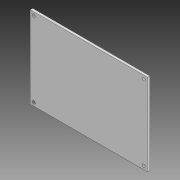
# Autodesk Inventor part: Motherboard
Saved by Autodesk Inventor 2020 (Build 240168000, 168)
## iProperties
Created: 2021-06-02
Part Number: Motherboard
Material: Generic
Document SubType Name: Modeling
Designer: DDeGo
Density: 1 g/cm^3
Appearance: Default
Author: DDeGo
Autodesk Inventor part; units mm, degrees
ref_plane "YZ Plane" through (0, 0, 0) normal (1, 0, 0) x (0, 1, 0)
ref_plane "XZ Plane" through (0, 0, 0) normal (0, 1, 0) x (-1, 0, 0)
ref_plane "XY Plane" through (0, 0, 0) normal (0, 0, 1) x (1, 0, 0)
sketch "Sketch1" plane through (0, 0, 0) normal (0, 0, 1) x (1, 0, 0)
  line L0 (-50, -35) -> (50, -35)
  line L1 (50, -35) -> (50, 35)
  line L2 (50, 35) -> (-50, 35)
  line L3 (-50, 35) -> (-50, -35)
  line L4 (-50, -35) -> (50, 35) construction
  line L5 (50, -35) -> (-50, 35) construction
  line L6 (47, -32) -> (-47, -32) construction
  line L7 (-47, -32) -> (-47, 32) construction
  line L8 (-47, 32) -> (47, 32) construction
  line L9 (47, 32) -> (47, -32) construction
  line L10 (47, -32) -> (-47, 32) construction
  line L11 (-47, -32) -> (47, 32) construction
  circle A0 centre (-47, 32) radius 1.25
  circle A1 centre (-47, -32) radius 1.25
  circle A2 centre (47, -32) radius 1.25
  circle A3 centre (47, 32) radius 1.25
  point P0 (0, 0)
  dimension "d0" = 100
  dimension "d1" = 70
  dimension "d4" = 64
  dimension "d5" = 94
  dimension "d6" = 2.5
  constraints: 24 end point, 4 centre point, 4 coincident, 4 midpoint, 4 parallel, 3 equal radius, 2 horizontal, 2 perpendicular
  measures "d0" distance of L1.end L2.end
  measures "d1" distance of L0.end L1.end
  measures "d4" distance of L8.end L6.start
  measures "d5" distance of L7.end L8.end
  measures "d6" diameter of A0
extrude "Extrusion1" add sketch "Sketch1" along normal blind 2
body "Solid1"
